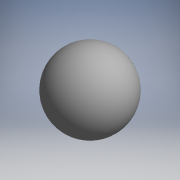
# Autodesk Inventor part: 6001JRX Ball
Saved by Autodesk Inventor 2017.3 (Build 213256000, 256)
## iProperties
Part Number: 6001JRX Ball
Material: Generic
Catalog Web Link: www.cadenas.de
Description: Open type ball-Deep Groove Ball Bearings
Vendor: NTN
Document SubType Name: Modeling
Designer: partserver
Manufacturer: NTN
Mass: 0.0550585 g
Surface Area: 0.699897 cm^2
Volume: 0.0550585 cm^3
Density: 1 g/cm^3
Appearance: PSOLRGB-192-192-192
Category: PARTsolutions
Company: NTN
Title: 6001JRX Ball
Author: Cadenas PARTsolutions
Comments: Deep Groove Ball Bearings
PSOL_IDENT_0: {$CADENAS_DATA\23d-libs\ntn\ball_roller_bearings\deep_groove_bb\deep_groove_bb\6_types\dgbb_ball.prj
PSOL_IDENT_1: },174 {VTYP=3D},{NB=6001JRX Ball},{LINA=6001JRX Ball},{NN=Open type ball},{DATE=12.08.2020 02:23:39}
PSOL_IDENT_2: ,{GEOMDATE=13.03.2020 06:49:14},{VERSION=},{LINEID=8980},{WBVAR=},{WBNUMERIC=}  {NB=6001JRX Ball},{L
PSOL_IDENT_3: INA=6001JRX Ball},{KT=DUMMY},{IDNR=},{SD=12},{D=28},{B=8},{R=0.3},{ORDER1=6001JRX},{ORDER=6001JRX},{
PSOL_IDENT_4: CR=5.65},{COR=2.39},{CRF=MIN},{CORF=MIN},{LSG=26000},{LSO=30000},{MASS=0.021},{RNS=MIN},{LLH=MIN},{L
PSOL_IDENT_5: LU=MIN},{ST=},{NCST=},{LTST=},{CST=},{SRG=},{SR=},{D1=26.44},{A=2.20},{BA=0.90},{R0=0.30},{D2=32.7},
PSOL_IDENT_6: {F=MIN},{DA1=},{DA2=},{DA=},{DX=MIN},{CY=},{CZ=},{RAS=},{RNAS=},{VERS=1},{X=8}
NB: 6001JRX Ball
NN: Open type ball
NT: Deep Groove Ball Bearings
NBSYN: $ORDER. Ball
LINA: 6001JRX Ball
CATALOG: NTN Corporation
SD: 12
D: 28
B: 8
R: 0.3
ORDER1: 6001JRX
ORDER: 6001JRX
CR: 5.65
COR: 2.39
CRF: 0
CORF: 0
LSG: 26000
LSO: 30000
MASS: 0.021
RNS: 0
LLH: 0
LLU: 0
D1: 26.44
A: 2.2
BA: 0.9
R0: 0.3
D2: 32.7
F: 0
DX: 0
VERS: 1
SUPPLIER: NTN
ARTICLENO: 6001JRX Ball
BOMINFO: 6001JRX Ball
CREATOR: CADENAS GmbH
Autodesk Inventor part; units mm, degrees
sketch "Sketch_1" plane through (0, 0, 0) normal (0, 0, 1) x (1, 0, 0)
  line L0 (2.36, 0) -> (-2.36, 0)
  arc A0 (2.36, 0) -> (-2.36, 0) centre (0, 0) ccw
  line L1 (2.36, 0) -> (-2.36, 0)
  constraints: 4 end point, 2 point on circle, 1 centre point
revolve "Revolution1" add sketch "Sketch_1" angle 360 about axis through (2.36, 0, 0) along (1, 0, 0)
ref_plane "dgbb_ball_XY" through (0, 0, 0) normal (1, 0, 0) x (0, 0, -1)
ref_plane "dgbb_ball_YZ" through (0, 0, 0) normal (0, 0, -1) x (0, 1, 0)
ref_plane "dgbb_ball_ZX" through (0, 0, 0) normal (0, 1, 0) x (1, 0, 0)
body "Solid1"
